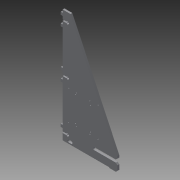
# Autodesk Inventor part: support2_import
Saved by Autodesk Inventor 2015 (Build 190159000, 159)
## iProperties
Created: 2015-04-20
Part Number: support2_import
Material: Generic
Document SubType Name: Modeling
Designer: X
Density: 1 g/cm^3
Appearance: Default
Author: X
Autodesk Inventor part; units mm, degrees
ref_plane "YZ Plane" through (0, 0, 0) normal (1, 0, 0) x (0, 1, 0)
ref_plane "XZ Plane" through (0, 0, 0) normal (0, 1, 0) x (-1, 0, 0)
ref_plane "XY Plane" through (0, 0, 0) normal (0, 0, 1) x (1, 0, 0)
sketch "Sketch1" plane through (0, 0, 0) normal (0, 1, 0) x (-1, 0, 0)
  line L0 (260.0009, -122.7811) -> (259.5668, -122.6012)
  line L1 (259.5668, -122.6012) -> (259.1941, -122.3151)
  line L2 (259.1941, -122.3151) -> (258.9081, -121.9423)
  line L3 (258.9081, -121.9423) -> (258.7283, -121.5081)
  line L4 (258.7283, -121.5081) -> (258.6671, -121.0423)
  line L5 (258.6671, -121.0423) -> (258.7285, -120.5764)
  line L6 (258.7285, -120.5764) -> (258.9084, -120.1423)
  line L7 (258.9084, -120.1423) -> (259.1945, -119.7695)
  line L8 (259.1945, -119.7695) -> (259.5673, -119.4835)
  line L9 (259.5673, -119.4835) -> (260.0014, -119.3038)
  line L10 (260.0014, -119.3038) -> (260.4673, -119.2425)
  line L11 (260.4673, -119.2425) -> (260.9332, -119.3039)
  line L12 (260.9332, -119.3039) -> (261.3673, -119.4838)
  line L13 (261.3673, -119.4838) -> (261.74, -119.7699)
  line L14 (261.74, -119.7699) -> (262.026, -120.1427)
  line L15 (262.026, -120.1427) -> (262.2058, -120.5769)
  line L16 (262.2058, -120.5769) -> (262.2671, -121.0428)
  line L17 (262.2671, -121.0428) -> (262.2057, -121.5086)
  line L18 (262.2057, -121.5086) -> (262.0258, -121.9427)
  line L19 (262.0258, -121.9427) -> (261.7397, -122.3155)
  line L20 (261.7397, -122.3155) -> (261.3668, -122.6015)
  line L21 (261.3668, -122.6015) -> (260.9327, -122.7812)
  line L22 (260.9327, -122.7812) -> (260.4668, -122.8425)
  line L23 (260.4668, -122.8425) -> (260.0009, -122.7811)
  line L24 (218.2738, -121.5086) -> (218.0939, -121.9427)
  line L25 (218.0939, -121.9427) -> (217.8078, -122.3155)
  line L26 (217.8078, -122.3155) -> (217.4349, -122.6015)
  line L27 (217.4349, -122.6015) -> (217.0008, -122.7812)
  line L28 (217.0008, -122.7812) -> (216.5349, -122.8425)
  line L29 (216.5349, -122.8425) -> (216.069, -122.7811)
  line L30 (216.069, -122.7811) -> (215.6349, -122.6012)
  line L31 (215.6349, -122.6012) -> (215.2622, -122.3151)
  line L32 (215.2622, -122.3151) -> (214.9762, -121.9423)
  line L33 (214.9762, -121.9423) -> (214.7964, -121.5081)
  line L34 (214.7964, -121.5081) -> (214.7352, -121.0423)
  line L35 (214.7352, -121.0423) -> (214.7966, -120.5764)
  line L36 (214.7966, -120.5764) -> (214.9765, -120.1423)
  line L37 (214.9765, -120.1423) -> (215.2626, -119.7695)
  line L38 (215.2626, -119.7695) -> (215.6354, -119.4835)
  line L39 (215.6354, -119.4835) -> (216.0695, -119.3038)
  line L40 (216.0695, -119.3038) -> (216.5354, -119.2425)
  line L41 (216.5354, -119.2425) -> (217.0013, -119.3039)
  line L42 (217.0013, -119.3039) -> (217.4354, -119.4838)
  line L43 (217.4354, -119.4838) -> (217.8081, -119.7699)
  line L44 (217.8081, -119.7699) -> (218.0941, -120.1427)
  line L45 (218.0941, -120.1427) -> (218.2739, -120.5769)
  line L46 (218.2739, -120.5769) -> (218.3352, -121.0428)
  line L47 (218.3352, -121.0428) -> (218.2738, -121.5086)
  line L48 (260.4348, -28.8258) -> (259.9689, -28.7644)
  line L49 (259.9689, -28.7644) -> (259.5348, -28.5846)
  line L50 (259.5348, -28.5846) -> (259.1621, -28.2985)
  line L51 (259.1621, -28.2985) -> (258.8761, -27.9256)
  line L52 (258.8761, -27.9256) -> (258.6963, -27.4915)
  line L53 (258.6963, -27.4915) -> (258.635, -27.0256)
  line L54 (258.635, -27.0256) -> (258.6964, -26.5597)
  line L55 (258.6964, -26.5597) -> (258.8763, -26.1256)
  line L56 (258.8763, -26.1256) -> (259.1624, -25.7529)
  line L57 (259.1624, -25.7529) -> (259.5353, -25.4669)
  line L58 (259.5353, -25.4669) -> (259.9694, -25.2871)
  line L59 (259.9694, -25.2871) -> (260.4353, -25.2258)
  line L60 (260.4353, -25.2258) -> (260.9012, -25.2872)
  line L61 (260.9012, -25.2872) -> (261.3353, -25.4671)
  line L62 (261.3353, -25.4671) -> (261.708, -25.7532)
  line L63 (261.708, -25.7532) -> (261.994, -26.1261)
  line L64 (261.994, -26.1261) -> (262.1738, -26.5602)
  line L65 (262.1738, -26.5602) -> (262.235, -27.0261)
  line L66 (262.235, -27.0261) -> (262.1736, -27.492)
  line L67 (262.1736, -27.492) -> (261.9938, -27.9261)
  line L68 (261.9938, -27.9261) -> (261.7076, -28.2988)
  line L69 (261.7076, -28.2988) -> (261.3348, -28.5848)
  line L70 (261.3348, -28.5848) -> (260.9007, -28.7646)
  line L71 (260.9007, -28.7646) -> (260.4348, -28.8258)
  line L72 (218.1596, -28.0183) -> (217.8734, -28.391)
  line L73 (217.8734, -28.391) -> (217.5006, -28.677)
  line L74 (217.5006, -28.677) -> (217.0665, -28.8568)
  line L75 (217.0665, -28.8568) -> (216.6006, -28.9181)
  line L76 (216.6006, -28.9181) -> (216.1347, -28.8567)
  line L77 (216.1347, -28.8567) -> (215.7006, -28.6768)
  line L78 (215.7006, -28.6768) -> (215.3279, -28.3907)
  line L79 (215.3279, -28.3907) -> (215.0419, -28.0178)
  line L80 (215.0419, -28.0178) -> (214.8621, -27.5837)
  line L81 (214.8621, -27.5837) -> (214.8008, -27.1178)
  line L82 (214.8008, -27.1178) -> (214.8622, -26.6519)
  line L83 (214.8622, -26.6519) -> (215.0421, -26.2178)
  line L84 (215.0421, -26.2178) -> (215.3282, -25.8451)
  line L85 (215.3282, -25.8451) -> (215.7011, -25.5591)
  line L86 (215.7011, -25.5591) -> (216.1352, -25.3793)
  line L87 (216.1352, -25.3793) -> (216.6011, -25.3181)
  line L88 (216.6011, -25.3181) -> (217.067, -25.3795)
  line L89 (217.067, -25.3795) -> (217.5011, -25.5593)
  line L90 (217.5011, -25.5593) -> (217.8738, -25.8455)
  line L91 (217.8738, -25.8455) -> (218.1598, -26.2183)
  line L92 (218.1598, -26.2183) -> (218.3396, -26.6524)
  line L93 (218.3396, -26.6524) -> (218.4008, -27.1183)
  line L94 (218.4008, -27.1183) -> (218.3394, -27.5842)
  line L95 (218.3394, -27.5842) -> (218.1596, -28.0183)
  line L96 (262.1401, -115.7635) -> (261.9604, -115.6735)
  line L97 (261.9604, -115.6735) -> (261.706, -115.5836)
  line L98 (261.706, -115.5836) -> (261.3333, -115.2975)
  line L99 (261.3333, -115.2975) -> (261.0473, -114.9247)
  line L100 (261.0473, -114.9247) -> (260.8675, -114.4906)
  line L101 (260.8675, -114.4906) -> (260.8063, -114.0247)
  line L102 (260.8063, -114.0247) -> (260.8677, -113.5588)
  line L103 (260.8677, -113.5588) -> (261.0475, -113.1247)
  line L104 (261.0475, -113.1247) -> (261.3336, -112.752)
  line L105 (261.3336, -112.752) -> (261.7065, -112.466)
  line L106 (261.7065, -112.466) -> (262.1406, -112.2862)
  line L107 (262.1406, -112.2862) -> (262.6065, -112.2249)
  line L108 (262.6065, -112.2249) -> (263.0724, -112.2863)
  line L109 (263.0724, -112.2863) -> (263.2717, -112.3689)
  line L110 (263.2717, -112.3689) -> (263.3268, -112.3762)
  line L111 (263.3268, -112.3762) -> (263.5065, -112.4662)
  line L112 (263.5065, -112.4662) -> (263.8792, -112.7523)
  line L113 (263.8792, -112.7523) -> (264.1652, -113.1252)
  line L114 (264.1652, -113.1252) -> (264.345, -113.5593)
  line L115 (264.345, -113.5593) -> (264.4063, -114.0252)
  line L116 (264.4063, -114.0252) -> (264.3449, -114.4911)
  line L117 (264.3449, -114.4911) -> (264.165, -114.9252)
  line L118 (264.165, -114.9252) -> (263.8789, -115.2979)
  line L119 (263.8789, -115.2979) -> (263.506, -115.5839)
  line L120 (263.506, -115.5839) -> (263.0719, -115.7637)
  line L121 (263.0719, -115.7637) -> (262.606, -115.8249)
  line L122 (262.606, -115.8249) -> (262.1401, -115.7635)
  line L123 (263.8493, -31.4356) -> (264.1353, -31.8084)
  line L124 (264.1353, -31.8084) -> (264.315, -32.2426)
  line L125 (264.315, -32.2426) -> (264.3763, -32.7085)
  line L126 (264.3763, -32.7085) -> (264.3149, -33.1743)
  line L127 (264.3149, -33.1743) -> (264.135, -33.6084)
  line L128 (264.135, -33.6084) -> (263.8489, -33.9812)
  line L129 (263.8489, -33.9812) -> (263.4761, -34.2672)
  line L130 (263.4761, -34.2672) -> (263.0419, -34.447)
  line L131 (263.0419, -34.447) -> (262.576, -34.5082)
  line L132 (262.576, -34.5082) -> (262.1102, -34.4468)
  line L133 (262.1102, -34.4468) -> (261.6761, -34.2669)
  line L134 (261.6761, -34.2669) -> (261.5253, -34.1252)
  line L135 (261.5253, -34.1252) -> (261.3033, -33.9808)
  line L136 (261.3033, -33.9808) -> (261.0173, -33.608)
  line L137 (261.0173, -33.608) -> (260.8375, -33.1738)
  line L138 (260.8375, -33.1738) -> (260.7763, -32.708)
  line L139 (260.7763, -32.708) -> (260.8377, -32.2421)
  line L140 (260.8377, -32.2421) -> (261.0176, -31.808)
  line L141 (261.0176, -31.808) -> (261.3037, -31.4352)
  line L142 (261.3037, -31.4352) -> (261.6765, -31.1492)
  line L143 (261.6765, -31.1492) -> (262.1107, -30.9695)
  line L144 (262.1107, -30.9695) -> (262.5765, -30.9082)
  line L145 (262.5765, -30.9082) -> (263.0424, -30.9696)
  line L146 (263.0424, -30.9696) -> (263.4765, -31.1495)
  line L147 (263.4765, -31.1495) -> (263.6248, -31.2634)
  line L148 (263.6248, -31.2634) -> (263.6985, -31.2939)
  line L149 (263.6985, -31.2939) -> (263.8493, -31.4356)
  line L150 (213.0731, -115.226) -> (212.7871, -114.8532)
  line L151 (212.7871, -114.8532) -> (212.6073, -114.4191)
  line L152 (212.6073, -114.4191) -> (212.546, -113.9532)
  line L153 (212.546, -113.9532) -> (212.6074, -113.4873)
  line L154 (212.6074, -113.4873) -> (212.7873, -113.0532)
  line L155 (212.7873, -113.0532) -> (213.0734, -112.6805)
  line L156 (213.0734, -112.6805) -> (213.4463, -112.3945)
  line L157 (213.4463, -112.3945) -> (213.8804, -112.2147)
  line L158 (213.8804, -112.2147) -> (214.3463, -112.1534)
  line L159 (214.3463, -112.1534) -> (214.8122, -112.2148)
  line L160 (214.8122, -112.2148) -> (215.2463, -112.3947)
  line L161 (215.2463, -112.3947) -> (215.3565, -112.4793)
  line L162 (215.3565, -112.4793) -> (215.4311, -112.5103)
  line L163 (215.4311, -112.5103) -> (215.619, -112.6808)
  line L164 (215.619, -112.6808) -> (215.905, -113.0537)
  line L165 (215.905, -113.0537) -> (216.0848, -113.4878)
  line L166 (216.0848, -113.4878) -> (216.146, -113.9537)
  line L167 (216.146, -113.9537) -> (216.0846, -114.4196)
  line L168 (216.0846, -114.4196) -> (215.9048, -114.8537)
  line L169 (215.9048, -114.8537) -> (215.6187, -115.2264)
  line L170 (215.6187, -115.2264) -> (215.2458, -115.5124)
  line L171 (215.2458, -115.5124) -> (214.8117, -115.6922)
  line L172 (214.8117, -115.6922) -> (214.3458, -115.7534)
  line L173 (214.3458, -115.7534) -> (213.8799, -115.692)
  line L174 (213.8799, -115.692) -> (213.4458, -115.5121)
  line L175 (213.4458, -115.5121) -> (213.2579, -115.3416)
  line L176 (213.2579, -115.3416) -> (213.0731, -115.226)
  line L177 (215.4761, -37.6349) -> (215.5861, -37.7363)
  line L178 (215.5861, -37.7363) -> (215.8721, -38.1091)
  line L179 (215.8721, -38.1091) -> (216.0518, -38.5433)
  line L180 (216.0518, -38.5433) -> (216.1131, -39.0092)
  line L181 (216.1131, -39.0092) -> (216.0517, -39.475)
  line L182 (216.0517, -39.475) -> (215.8718, -39.9091)
  line L183 (215.8718, -39.9091) -> (215.5857, -40.2819)
  line L184 (215.5857, -40.2819) -> (215.2129, -40.5679)
  line L185 (215.2129, -40.5679) -> (214.7787, -40.7476)
  line L186 (214.7787, -40.7476) -> (214.3128, -40.8089)
  line L187 (214.3128, -40.8089) -> (213.847, -40.7475)
  line L188 (213.847, -40.7475) -> (213.4129, -40.5676)
  line L189 (213.4129, -40.5676) -> (213.3029, -40.4663)
  line L190 (213.3029, -40.4663) -> (213.0401, -40.2815)
  line L191 (213.0401, -40.2815) -> (212.7541, -39.9087)
  line L192 (212.7541, -39.9087) -> (212.5744, -39.4745)
  line L193 (212.5744, -39.4745) -> (212.5131, -39.0086)
  line L194 (212.5131, -39.0086) -> (212.5745, -38.5428)
  line L195 (212.5745, -38.5428) -> (212.7544, -38.1087)
  line L196 (212.7544, -38.1087) -> (213.0405, -37.7359)
  line L197 (213.0405, -37.7359) -> (213.4133, -37.4499)
  line L198 (213.4133, -37.4499) -> (213.8475, -37.2702)
  line L199 (213.8475, -37.2702) -> (214.3134, -37.2089)
  line L200 (214.3134, -37.2089) -> (214.7792, -37.2703)
  line L201 (214.7792, -37.2703) -> (215.2133, -37.4502)
  line L202 (215.2133, -37.4502) -> (215.4281, -37.6151)
  line L203 (215.4281, -37.6151) -> (215.4761, -37.6349)
  line L204 (286.7385, -25.8534) -> (286.6771, -26.3192)
  line L205 (286.6771, -26.3192) -> (286.4972, -26.7533)
  line L206 (286.4972, -26.7533) -> (286.2111, -27.1261)
  line L207 (286.2111, -27.1261) -> (285.8383, -27.4121)
  line L208 (285.8383, -27.4121) -> (285.4041, -27.5919)
  line L209 (285.4041, -27.5919) -> (284.9382, -27.6531)
  line L210 (284.9382, -27.6531) -> (284.4724, -27.5917)
  line L211 (284.4724, -27.5917) -> (284.0383, -27.4118)
  line L212 (284.0383, -27.4118) -> (283.6655, -27.1257)
  line L213 (283.6655, -27.1257) -> (283.3795, -26.7529)
  line L214 (283.3795, -26.7529) -> (283.1997, -26.3187)
  line L215 (283.1997, -26.3187) -> (283.1385, -25.8529)
  line L216 (283.1385, -25.8529) -> (283.1999, -25.387)
  line L217 (283.1999, -25.387) -> (283.3798, -24.9529)
  line L218 (283.3798, -24.9529) -> (283.6659, -24.5801)
  line L219 (283.6659, -24.5801) -> (284.0387, -24.2941)
  line L220 (284.0387, -24.2941) -> (284.4729, -24.1144)
  line L221 (284.4729, -24.1144) -> (284.9387, -24.0531)
  line L222 (284.9387, -24.0531) -> (285.4046, -24.1145)
  line L223 (285.4046, -24.1145) -> (285.8387, -24.2944)
  line L224 (285.8387, -24.2944) -> (286.2115, -24.5805)
  line L225 (286.2115, -24.5805) -> (286.4975, -24.9533)
  line L226 (286.4975, -24.9533) -> (286.6772, -25.3875)
  line L227 (286.6772, -25.3875) -> (286.7385, -25.8534)
  line L228 (191.5284, -120.8663) -> (191.7081, -121.3004)
  line L229 (191.7081, -121.3004) -> (191.7694, -121.7663)
  line L230 (191.7694, -121.7663) -> (191.708, -122.2322)
  line L231 (191.708, -122.2322) -> (191.5281, -122.6663)
  line L232 (191.5281, -122.6663) -> (191.242, -123.039)
  line L233 (191.242, -123.039) -> (190.8692, -123.325)
  line L234 (190.8692, -123.325) -> (190.435, -123.5048)
  line L235 (190.435, -123.5048) -> (189.9691, -123.566)
  line L236 (189.9691, -123.566) -> (189.5033, -123.5046)
  line L237 (189.5033, -123.5046) -> (189.0692, -123.3247)
  line L238 (189.0692, -123.3247) -> (188.6964, -123.0386)
  line L239 (188.6964, -123.0386) -> (188.4104, -122.6658)
  line L240 (188.4104, -122.6658) -> (188.2307, -122.2317)
  line L241 (188.2307, -122.2317) -> (188.1694, -121.7658)
  line L242 (188.1694, -121.7658) -> (188.2308, -121.2999)
  line L243 (188.2308, -121.2999) -> (188.4107, -120.8658)
  line L244 (188.4107, -120.8658) -> (188.6968, -120.4931)
  line L245 (188.6968, -120.4931) -> (189.0696, -120.2071)
  line L246 (189.0696, -120.2071) -> (189.5038, -120.0273)
  line L247 (189.5038, -120.0273) -> (189.9697, -119.966)
  line L248 (189.9697, -119.966) -> (190.4355, -120.0274)
  line L249 (190.4355, -120.0274) -> (190.8696, -120.2073)
  line L250 (190.8696, -120.2073) -> (191.2424, -120.4934)
  line L251 (191.2424, -120.4934) -> (191.5284, -120.8663)
  line L252 (283.4035, -122.7094) -> (283.2237, -122.2752)
  line L253 (283.2237, -122.2752) -> (283.1625, -121.8093)
  line L254 (283.1625, -121.8093) -> (283.2239, -121.3435)
  line L255 (283.2239, -121.3435) -> (283.4038, -120.9094)
  line L256 (283.4038, -120.9094) -> (283.6899, -120.5366)
  line L257 (283.6899, -120.5366) -> (284.0627, -120.2506)
  line L258 (284.0627, -120.2506) -> (284.4968, -120.0709)
  line L259 (284.4968, -120.0709) -> (284.9627, -120.0096)
  line L260 (284.9627, -120.0096) -> (285.4286, -120.071)
  line L261 (285.4286, -120.071) -> (285.8627, -120.2509)
  line L262 (285.8627, -120.2509) -> (286.2354, -120.537)
  line L263 (286.2354, -120.537) -> (286.5214, -120.9098)
  line L264 (286.5214, -120.9098) -> (286.7012, -121.344)
  line L265 (286.7012, -121.344) -> (286.7625, -121.8099)
  line L266 (286.7625, -121.8099) -> (286.7011, -122.2757)
  line L267 (286.7011, -122.2757) -> (286.5212, -122.7098)
  line L268 (286.5212, -122.7098) -> (286.2351, -123.0826)
  line L269 (286.2351, -123.0826) -> (285.8622, -123.3686)
  line L270 (285.8622, -123.3686) -> (285.4281, -123.5483)
  line L271 (285.4281, -123.5483) -> (284.9622, -123.6096)
  line L272 (284.9622, -123.6096) -> (284.4963, -123.5482)
  line L273 (284.4963, -123.5482) -> (284.0622, -123.3683)
  line L274 (284.0622, -123.3683) -> (283.6895, -123.0822)
  line L275 (283.6895, -123.0822) -> (283.4035, -122.7094)
  line L276 (191.7452, -25.899) -> (191.6838, -26.3649)
  line L277 (191.6838, -26.3649) -> (191.5039, -26.799)
  line L278 (191.5039, -26.799) -> (191.2178, -27.1717)
  line L279 (191.2178, -27.1717) -> (190.845, -27.4577)
  line L280 (190.845, -27.4577) -> (190.4108, -27.6375)
  line L281 (190.4108, -27.6375) -> (189.9449, -27.6988)
  line L282 (189.9449, -27.6988) -> (189.4791, -27.6374)
  line L283 (189.4791, -27.6374) -> (189.045, -27.4575)
  line L284 (189.045, -27.4575) -> (188.6722, -27.1714)
  line L285 (188.6722, -27.1714) -> (188.3862, -26.7985)
  line L286 (188.3862, -26.7985) -> (188.2065, -26.3644)
  line L287 (188.2065, -26.3644) -> (188.1452, -25.8985)
  line L288 (188.1452, -25.8985) -> (188.2066, -25.4326)
  line L289 (188.2066, -25.4326) -> (188.3865, -24.9985)
  line L290 (188.3865, -24.9985) -> (188.6726, -24.6258)
  line L291 (188.6726, -24.6258) -> (189.0454, -24.3398)
  line L292 (189.0454, -24.3398) -> (189.4796, -24.16)
  line L293 (189.4796, -24.16) -> (189.9455, -24.0988)
  line L294 (189.9455, -24.0988) -> (190.4113, -24.1602)
  line L295 (190.4113, -24.1602) -> (190.8454, -24.3401)
  line L296 (190.8454, -24.3401) -> (191.2182, -24.6262)
  line L297 (191.2182, -24.6262) -> (191.5042, -24.999)
  line L298 (191.5042, -24.999) -> (191.6839, -25.4331)
  line L299 (191.6839, -25.4331) -> (191.7452, -25.899)
  line L300 (272.4385, -175.0318) -> (272.5748, -173.9965)
  line L301 (272.5748, -173.9965) -> (272.9744, -173.0318)
  line L302 (272.9744, -173.0318) -> (273.6101, -172.2034)
  line L303 (273.6101, -172.2034) -> (274.4385, -171.5677)
  line L304 (274.4385, -171.5677) -> (275.4032, -171.1681)
  line L305 (275.4032, -171.1681) -> (276.4385, -171.0318)
  line L306 (276.4385, -171.0318) -> (284.4345, -171.0318)
  line L307 (284.4345, -171.0318) -> (285.4697, -171.1681)
  line L308 (285.4697, -171.1681) -> (286.4345, -171.5677)
  line L309 (286.4345, -171.5677) -> (287.2629, -172.2034)
  line L310 (287.2629, -172.2034) -> (287.8986, -173.0318)
  line L311 (287.8986, -173.0318) -> (288.2982, -173.9965)
  line L312 (288.2982, -173.9965) -> (288.4345, -175.0318)
  line L313 (288.4345, -175.0318) -> (288.2982, -176.0671)
  line L314 (288.2982, -176.0671) -> (287.8986, -177.0318)
  line L315 (287.8986, -177.0318) -> (287.2629, -177.8603)
  line L316 (287.2629, -177.8603) -> (286.4345, -178.4959)
  line L317 (286.4345, -178.4959) -> (285.4697, -178.8955)
  line L318 (285.4697, -178.8955) -> (284.4345, -179.0318)
  line L319 (284.4345, -179.0318) -> (276.3716, -179.0318)
  line L320 (276.3716, -179.0318) -> (275.4032, -178.8955)
  line L321 (275.4032, -178.8955) -> (274.4385, -178.4959)
  line L322 (274.4385, -178.4959) -> (273.6101, -177.8603)
  line L323 (273.6101, -177.8603) -> (272.9744, -177.0318)
  line L324 (272.9744, -177.0318) -> (272.5748, -176.0671)
  line L325 (272.5748, -176.0671) -> (272.4385, -175.0318)
  line L326 (201.5714, -159.4318) -> (131.5714, -159.4318)
  line L327 (131.5714, -159.4318) -> (126.5714, -164.4318)
  line L328 (126.5714, -164.4318) -> (126.5714, -180.0318)
  line L329 (126.5714, -180.0318) -> (131.5714, -185.0318)
  line L330 (131.5714, -185.0318) -> (151.5714, -185.0318)
  line L331 (151.5714, -185.0318) -> (153.5714, -183.0318)
  line L332 (153.5714, -183.0318) -> (304.3714, -183.0318)
  line L333 (304.3714, -183.0318) -> (304.3714, -162.2374)
  line L334 (304.3714, -162.2374) -> (292.3714, -162.2374)
  line L335 (292.3714, -162.2374) -> (292.3714, -164.0374)
  line L336 (292.3714, -164.0374) -> (287.2714, -164.0374)
  line L337 (287.2714, -164.0374) -> (287.2714, -162.2374)
  line L338 (287.2714, -162.2374) -> (283.2714, -162.2374)
  line L339 (283.2714, -162.2374) -> (283.2714, -157.8374)
  line L340 (283.2714, -157.8374) -> (287.2714, -157.8374)
  line L341 (287.2714, -157.8374) -> (287.2714, -156.0374)
  line L342 (287.2714, -156.0374) -> (292.3714, -156.0374)
  line L343 (292.3714, -156.0374) -> (292.3714, -157.8374)
  line L344 (292.3714, -157.8374) -> (304.3714, -157.8374)
  line L345 (304.3714, -157.8374) -> (304.3714, -148.2819)
  line L346 (304.3714, -148.2819) -> (310.4714, -148.2819)
  line L347 (310.4714, -148.2819) -> (310.4714, -139.4819)
  line L348 (310.4714, -139.4819) -> (304.3714, -139.4819)
  line L349 (304.3714, -139.4819) -> (304.3714, -20.5818)
  line L350 (304.3714, -20.5818) -> (310.4714, -20.5818)
  line L351 (310.4714, -20.5818) -> (310.4714, -11.7818)
  line L352 (310.4714, -11.7818) -> (304.3714, -11.7818)
  line L353 (304.3714, -11.7818) -> (304.3714, -2.2318)
  line L354 (304.3714, -2.2318) -> (292.3714, -2.2318)
  line L355 (292.3714, -2.2318) -> (292.3714, -4.0318)
  line L356 (292.3714, -4.0318) -> (287.2714, -4.0318)
  line L357 (287.2714, -4.0318) -> (287.2714, -2.2318)
  line L358 (287.2714, -2.2318) -> (283.2714, -2.2318)
  line L359 (283.2714, -2.2318) -> (283.2714, 2.1682)
  line L360 (283.2714, 2.1682) -> (287.2714, 2.1682)
  line L361 (287.2714, 2.1682) -> (287.2714, 3.9682)
  line L362 (287.2714, 3.9682) -> (292.3714, 3.9682)
  line L363 (292.3714, 3.9682) -> (292.3714, 2.1682)
  line L364 (292.3714, 2.1682) -> (304.3714, 2.1682)
  line L365 (304.3714, 2.1682) -> (304.3714, 11.7182)
  line L366 (304.3714, 11.7182) -> (310.4714, 11.7182)
  line L367 (310.4714, 11.7182) -> (310.4714, 20.5182)
  line L368 (310.4714, 20.5182) -> (304.3714, 20.5182)
  line L369 (304.3714, 20.5182) -> (304.3714, 134.5109)
  line L370 (304.3714, 134.5109) -> (310.4714, 134.5109)
  line L371 (310.4714, 134.5109) -> (310.4714, 143.3109)
  line L372 (310.4714, 143.3109) -> (304.3714, 143.3109)
  line L373 (304.3714, 143.3109) -> (304.3714, 152.8531)
  line L374 (304.3714, 152.8531) -> (292.3714, 152.8531)
  line L375 (292.3714, 152.8531) -> (292.3714, 151.0531)
  line L376 (292.3714, 151.0531) -> (287.2714, 151.0531)
  line L377 (287.2714, 151.0531) -> (287.2714, 152.8531)
  line L378 (287.2714, 152.8531) -> (283.2714, 152.8531)
  line L379 (283.2714, 152.8531) -> (283.2714, 157.2531)
  line L380 (283.2714, 157.2531) -> (287.2714, 157.2531)
  line L381 (287.2714, 157.2531) -> (287.2714, 159.0531)
  line L382 (287.2714, 159.0531) -> (292.3714, 159.0531)
  line L383 (292.3714, 159.0531) -> (292.3714, 157.2531)
  line L384 (292.3714, 157.2531) -> (304.3714, 157.2531)
  line L385 (304.3714, 157.2531) -> (304.3714, 166.8109)
  line L386 (304.3714, 166.8109) -> (310.4714, 166.8109)
  line L387 (310.4714, 166.8109) -> (310.4714, 175.6109)
  line L388 (310.4714, 175.6109) -> (304.3714, 175.6109)
  line L389 (304.3714, 175.6109) -> (304.3714, 184.9681)
  line L390 (304.3714, 184.9681) -> (278.9714, 184.9681)
  line L391 (278.9714, 184.9681) -> (126.5714, -138.0318)
  line L392 (126.5714, -138.0318) -> (126.5714, -145.6318)
  line L393 (126.5714, -145.6318) -> (131.5714, -150.6318)
  line L394 (131.5714, -150.6318) -> (201.5714, -150.6318)
  line L395 (201.5714, -150.6318) -> (202.7102, -150.7818)
  line L396 (202.7102, -150.7818) -> (203.7714, -151.2213)
  line L397 (203.7714, -151.2213) -> (204.6826, -151.9206)
  line L398 (204.6826, -151.9206) -> (205.3819, -152.8318)
  line L399 (205.3819, -152.8318) -> (205.8214, -153.893)
  line L400 (205.8214, -153.893) -> (205.9714, -155.0318)
  line L401 (205.9714, -155.0318) -> (205.8214, -156.1706)
  line L402 (205.8214, -156.1706) -> (205.3819, -157.2318)
  line L403 (205.3819, -157.2318) -> (204.6826, -158.1431)
  line L404 (204.6826, -158.1431) -> (203.7714, -158.8423)
  line L405 (203.7714, -158.8423) -> (202.7102, -159.2819)
  line L406 (202.7102, -159.2819) -> (201.5714, -159.4318)
  constraints: 814 end point
extrude "Extrusion1" add sketch "Sketch1" along normal blind 6
body "Solid1"
